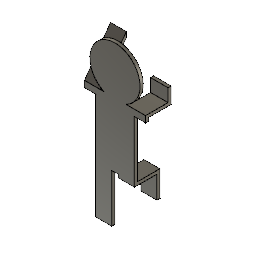
Rock Climber v1 (Autodesk Fusion 360 design; units mm, degrees)
Autodesk Fusion 360 part; units mm, degrees
sketch "Sketch1" plane through (0, 0, 0) normal (0, 1, 0) x (1, 0, 0)
  line L0 (0, 0) -> (5, 0)
  line L1 (5, 0) -> (5, -15)
  line L2 (5, -15) -> (0, -15)
  line L3 (0, -15) -> (0, 0)
  constraint horizontal L0
  constraint vertical L1
  constraint horizontal L2
  constraint vertical L3
  constraint coincident L0.start L3.end
extrude "Extrude1" add sketch "Sketch1" along normal blind 1
sketch "Sketch2" plane through (0, 0, 0) normal (0, -1, 0) x (1, 0, 0)
  line L0 (5, 15) -> (0, 15)
  line L1 (0, 15) -> (0, 0)
  line L2 (0, 0) -> (5, 0)
  line L3 (5, 0) -> (5, 15)
  line L4 (0, 15) -> (12, 15)
  line L5 (12, 15) -> (12, 35)
  line L6 (12, 35) -> (0, 35)
  line L7 (0, 35) -> (0, 15)
  constraint horizontal L4
  constraint vertical L5
  constraint horizontal L6
  constraint vertical L7
  constraint coincident L0.end L1.start
extrude "Extrude2" add sketch "Sketch2" against normal blind 1 contours L0 L4 L5 L6 L7
sketch "Sketch3" plane through (0, 0, 0) normal (0, 1, 0) x (1, 0, 0)
  line L0 (12, -15) -> (7, -15)
  line L1 (7, -15) -> (7, -14)
  line L2 (7, -14) -> (12, -14)
  line L3 (12, -14) -> (12, -15)
  constraint horizontal L0
  constraint vertical L1
  constraint horizontal L2
  constraint vertical L3
extrude "Extrude3" add sketch "Sketch3" along normal blind 8
sketch "Sketch4" plane through (0, 0, 14) normal (0, 0, -1) x (1, 0, 0)
  line L0 (12, 0) -> (7, 0)
  line L1 (7, 0) -> (7, -8)
  line L2 (7, -8) -> (12, -8)
  line L3 (12, -8) -> (12, 0)
  line L4 (7, -8) -> (12, -8)
  line L5 (12, -8) -> (12, -7)
  line L6 (12, -7) -> (7, -7)
  line L7 (7, -7) -> (7, -8)
  constraint horizontal L4
  constraint vertical L5
  constraint horizontal L6
  constraint vertical L7
  constraint coincident L3 L5.end
  constraint coincident L1.end L2.start
extrude "Extrude4" add sketch "Sketch4" along normal blind 7 contours L1 L2 L3 L4 L5 L6 L7
sketch "Sketch5" plane through (0, 0, 0) normal (0, 1, 0) x (1, 0, 0)
  circle A0 centre (6, -42) radius 7.8102
extrude "Extrude5" add sketch "Sketch5" along normal blind 1
sketch "Sketch6" plane through (0, 0, 0) normal (0, -1, 0) x (1, 0, 0)
  line L0 (2.5359, 35) -> (0, 35)
  line L1 (0, 35) -> (0, 0)
  line L2 (0, 0) -> (5, 0)
  line L3 (5, 0) -> (5, 15)
  line L4 (5, 15) -> (7, 15)
  line L5 (7, 15) -> (7, 14)
  line L6 (7, 14) -> (12, 14)
  line L7 (12, 14) -> (12, 35)
  line L8 (12, 35) -> (9.4641, 35)
  arc A0 (9.4641, 35) -> (2.5359, 35) centre (6, 42) ccw
  line L9 (-4.6664, 35.0926, -0.0359) -> (0.3336, 35.0926, -0.0359)
  line L10 (0.3336, 35.0926, -0.0359) -> (0.3336, 33.0926, -0.0359)
  line L11 (0.3336, 33.0926, -0.0359) -> (-4.6664, 33.0926, -0.0359)
  line L12 (-4.6664, 33.0926, -0.0359) -> (-4.6664, 35.0926, -0.0359)
  line L13 (6, 49.8103) -> (6, 20.3227)
  constraint midpoint A0 L13.start
  constraint vertical L13
extrude "Extrude6" add sketch "Sketch6" against normal blind 1 contours L9 L10 L11 L12 in plane through (0, 0.0359, 0) normal (0, -1, 0)
delete_face "DeleteFace1" 1 faces at (-3.1109, 0.0359, 34.3951)
sketch "Sketch7" plane through (0, 0, 0) normal (0, -1, 0) x (1, 0, 0)
  line L0 (2.5359, 35) -> (0, 35)
  line L1 (0, 35) -> (0, 0)
  line L2 (0, 0) -> (5, 0)
  line L3 (5, 0) -> (5, 15)
  line L4 (5, 15) -> (7, 15)
  line L5 (7, 15) -> (7, 14)
  line L6 (7, 14) -> (12, 14)
  line L7 (12, 14) -> (12, 35)
  line L8 (12, 35) -> (9.4641, 35)
  arc A0 (9.4641, 35) -> (2.5359, 35) centre (6, 42) ccw
  line L9 (-3.5, 35) -> (15.5, 35)
  line L10 (15.5, 35) -> (15.5, 33)
  line L11 (15.5, 33) -> (-3.5, 33)
  line L12 (-3.5, 33) -> (-3.5, 35)
  dimension "d13" = 2
  constraint horizontal L9
  constraint vertical L10
  constraint horizontal L11
  constraint vertical L12
  measures "d13" distance of L9 L11
extrude "Extrude7" add sketch "Sketch7" against normal blind 1 contours L0 L1 L7 L8 L9 L11 | L1 L9 L11 L12 | L7 L9 L10 L11
delete_face "DeleteFace2" 3 faces at (0.1112, 1.0359, 34.3642) (0, 1.012, 34.3642) (0.3336, 1.012, 34.3642)
sketch "Sketch8" plane through (0, 0, 0) normal (0, -1, 0) x (1, 0, 0)
  arc A0 (9.4641, 35) -> (2.5359, 35) centre (6, 42) ccw
  line L0 (2.5359, 35) -> (-3.5, 35)
  line L1 (-3.5, 35) -> (-3.5, 33)
  line L2 (-3.5, 33) -> (0, 33)
  line L3 (0, 33) -> (0, 0)
  line L4 (0, 0) -> (5, 0)
  line L5 (5, 0) -> (5, 15)
  line L6 (5, 15) -> (7, 15)
  line L7 (7, 15) -> (7, 14)
  line L8 (7, 14) -> (12, 14)
  line L9 (12, 14) -> (12, 33)
  line L10 (12, 33) -> (15.5, 33)
  line L11 (15.5, 33) -> (15.5, 35)
  line L12 (15.5, 35) -> (9.4641, 35)
  line L13 (-3.5, 35) -> (1.4633, 35)
  line L14 (1.4633, 35, 0) -> (1.4633, 49.0828, -9.8609)
  line L15 (1.4633, 49.0828, -9.8609) -> (-3.5, 49.0828, -9.8609)
  line L16 (-3.5, 49.0828, -9.8609) -> (-3.5, 35, 0)
  constraint coincident L0.end L1.start
extrude "Extrude8" add sketch "Sketch8" against normal blind 1 contours L0 L13 L14 L15 L16 in plane through (0, -16.4446, 11.5146) normal (0, -0.819152, 0.573576)
sketch "Sketch9" plane through (0, 0, 0) normal (0, -1, 0) x (1, 0, 0)
  arc A0 (9.4641, 35) -> (2.5359, 35) centre (6, 42) ccw
  line L0 (2.5359, 35) -> (1.4633, 35)
  line L1 (1.4633, 35) -> (-3.5, 35)
  line L2 (-3.5, 35) -> (-3.5, 33)
  line L3 (-3.5, 33) -> (0, 33)
  line L4 (0, 33) -> (0, 0)
  line L5 (0, 0) -> (5, 0)
  line L6 (5, 0) -> (5, 15)
  line L7 (5, 15) -> (7, 15)
  line L8 (7, 15) -> (7, 14)
  line L9 (7, 14) -> (12, 14)
  line L10 (12, 14) -> (12, 33)
  line L11 (12, 33) -> (15.5, 33)
  line L12 (15.5, 33) -> (15.5, 35)
  line L13 (15.5, 35) -> (9.4641, 35)
  line L14 (15.5, 35) -> (10, 35)
  line L15 (10, 35) -> (10, 34)
  line L16 (10, 34) -> (15.5, 34)
  line L17 (15.5, 34) -> (15.5, 35)
  constraint horizontal L14
  constraint vertical L15
  constraint horizontal L16
  constraint vertical L17
  constraint coincident L12.end L13.start
extrude "Extrude9" add sketch "Sketch9" against normal blind 8 contours L12 L13 L14 L15 L16 L17
sketch "Sketch10" plane through (0, 0, 35) normal (0, 0, 1) x (-1, 0, 0)
  line L0 (-10, -1) -> (-9.4641, -1)
  line L1 (-9.4641, -1) -> (-9.4641, 0)
  line L2 (-9.4641, 0) -> (-15.5, 0)
  line L3 (-15.5, 0) -> (-15.5, -8)
  line L4 (-15.5, -8) -> (-10, -8)
  line L5 (-10, -8) -> (-10, -1)
  line L6 (-10, -8) -> (-15.5, -8)
  line L7 (-15.5, -8) -> (-15.5, -7)
  line L8 (-15.5, -7) -> (-10, -7)
  line L9 (-10, -7) -> (-10, -8)
  constraint horizontal L6
  constraint vertical L7
  constraint horizontal L8
  constraint vertical L9
  constraint coincident L3 L7.end
  constraint coincident L4.end L5.start
extrude "Extrude10" add sketch "Sketch10" along normal blind 4 contours L3 L4 L5 L6 L7 L8 L9
sketch "Sketch11" plane through (0, 0, 0) normal (1, 0, 0) x (0, 1, 0)
  line L0 (8.105, -0.2879) -> (18.105, -0.2879)
  line L1 (18.105, -0.2879) -> (18.105, 54.7121)
  line L2 (18.105, 54.7121) -> (8.105, 54.7121)
  line L3 (8.105, 54.7121) -> (8.105, -0.2879)
  constraint horizontal L0
  constraint vertical L1
  constraint horizontal L2
  constraint vertical L3
extrude "Extrude11" cut sketch "Sketch11" along normal blind 20 and the other way blind 13
